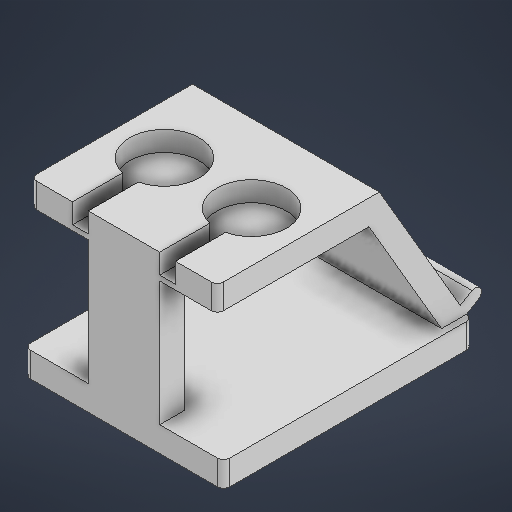
# Autodesk Inventor part: PhoneStand
Saved by Autodesk Inventor 2026.1 (Build 301233020, 233B)
## iProperties
Created: 2025-11-22
Part Number: PhoneStand
Material: Generic
Document SubType Name: Modeling
Designer: astro
Density: 1 g/cm^3
Appearance: Default
Author: astro
Autodesk Inventor part; units mm, degrees
ref_plane "YZ Plane" through (0, 0, 0) normal (1, 0, 0) x (0, 1, 0)
ref_plane "XZ Plane" through (0, 0, 0) normal (0, 1, 0) x (-1, 0, 0)
ref_plane "XY Plane" through (0, 0, 0) normal (0, 0, 1) x (1, 0, 0)
sketch "Sketch1" plane through (0, 0, 0) normal (0, 1, 0) x (-1, 0, 0)
  line L0 (-50.8, -63.5) -> (50.8, -63.5)
  line L1 (50.8, -63.5) -> (50.8, 63.5)
  line L2 (50.8, 63.5) -> (-50.8, 63.5)
  line L3 (-50.8, 63.5) -> (-50.8, -63.5)
  line L4 (-50.8, -63.5) -> (50.8, 63.5) construction
  line L5 (50.8, -63.5) -> (-50.8, 63.5) construction
  point P0 (0, 0)
  dimension "d0" = 101.6
  dimension "d1" = 127
  constraints: 12 end point, 2 midpoint, 2 parallel, 1 horizontal, 1 perpendicular
  measures "d0" distance of L2.end L1.end
  measures "d1" distance of L0.end L1.end
extrude "Extrusion1" add sketch "Sketch1" along normal blind 12.7
fillet "Fillet1" radius 3.175 4 edges at (-50.8, 6.35, 63.5) (50.8, 6.35, 63.5) (50.8, 6.35, -63.5) (-50.8, 6.35, -63.5)
sketch "Sketch2" plane through (0, 12.7, 0) normal (0, 1, 0) x (1, 0, 0)
  line L0 (47.625, 63.5) -> (-47.625, 63.5) projected
  line L1 (-47.625, 63.5) -> (47.625, 63.5)
  line L2 (47.625, 63.5) -> (47.625, 50.8)
  line L3 (47.625, 50.8) -> (-47.625, 50.8)
  line L4 (-47.625, 50.8) -> (-47.625, 63.5)
  line L5 (-47.625, -39.3448) -> (47.625, -39.3448)
  line L6 (47.625, -39.3448) -> (47.625, -60.325)
  line L7 (47.625, -60.325) -> (-47.625, -60.325)
  line L8 (-47.625, -60.325) -> (-47.625, -39.3448)
  point P0 (0, 0)
  dimension "d5" = 12.7
  constraints: 16 end point, 4 parallel, 2 horizontal, 2 perpendicular, 2 point on line
  measures "d5" distance of L1.end L2.end
extrude "Extrusion2" add sketch "Sketch2" along normal blind 76.2 contours L2 L3 L4 L0
sketch "Sketch3" plane through (47.625, 12.7, -50.8) normal (1, 0, 0) x (0, 0, -1)
  point P0 (-50.8, -12.7)
sketch "Sketch4" plane through (-47.625, 12.7, -50.8) normal (0, 0, 1) x (1, 0, 0)
  line L0 (0, 0) -> (0, 76.2) projected
  line L1 (95.25, 0) -> (98.425, 0) projected
  line L2 (0, 76.2) -> (95.25, 76.2)
  line L3 (95.25, 76.2) -> (95.25, 0)
  line L4 (95.25, 0) -> (0, 0)
  line L5 (0, 0) -> (0, 76.2)
  point P0 (47.625, -12.7)
  constraints: 8 end point, 2 parallel, 1 horizontal, 1 perpendicular
extrude "Extrusion3" add sketch "Sketch4" along normal blind 76.2
sketch "Sketch5" plane through (47.625, 12.7, -63.5) normal (1, 0, 0) x (0, 0, -1)
  line L0 (0, 76.2) -> (-88.9, 76.2) projected
  line L1 (0, 0) -> (0, 76.2) projected
  line L2 (-44.45, 76.2) -> (0, 0)
  line L3 (0, 0) -> (0, 76.2)
  line L4 (0, 76.2) -> (-44.45, 76.2)
  line L5 (0, 0) -> (-88.9, 0) projected
  line L6 (-88.9, 0) -> (-44.45, 76.2)
  line L7 (-88.9, 76.2) -> (-88.9, 0)
  line L8 (-88.9, 76.2) -> (-44.45, 76.2)
  point P0 (-63.5, -12.7)
  constraints: 12 end point, 3 perpendicular, 1 midpoint, 1 point on line
extrude "Extrusion4" cut sketch "Sketch5" against normal blind 95.25 contours L1 L2 L0
sketch "Sketch6" plane through (47.625, 12.7, 25.4) normal (1, 0, 0) x (0, 0, -1)
  line L0 (44.45, 76.2) -> (0, 76.2) projected
  line L1 (44.45, 76.2) -> (31.75, 76.2)
  line L2 (0, 0) -> (88.9, 0) projected
  line L3 (88.9, 0) -> (76.2, 0)
  line L4 (76.2, 0) -> (31.75, 76.2)
  line L5 (44.45, 76.2) -> (88.9, 0) projected
  line L6 (44.45, 76.2) -> (88.9, 0)
  line L7 (88.9, 0) -> (76.2, 0)
  line L8 (0, 76.2) -> (0, 0) projected
  line L9 (0, 76.2) -> (0, 0)
  line L10 (0, 0) -> (76.2, 0)
  line L11 (31.75, 76.2) -> (0, 76.2)
  point P0 (25.4, -12.7)
  dimension "d12" = 12.7
  dimension "d13" = 12.7
  constraints: 16 end point, 3 collinear, 2 point on line, 1 horizontal, 1 perpendicular
  measures "d12" distance of L0.start L1.end
  measures "d13" distance of L2.end L3.end
extrude "Extrusion5" cut sketch "Sketch6" against normal blind 95.25 contours L4 L2 L8 L0
sketch "Sketch7" plane through (-47.625, 12.7, -63.5) normal (-1, 0, 0) x (0, 0, 1)
  line L0 (44.45, 76.2) -> (57.15, 76.2) projected
  line L1 (127, -12.7) -> (127, 0) projected
  line L2 (57.15, 76.2) -> (127, 0)
  line L3 (57.15, 76.2) -> (127, 76.2)
  line L4 (127, 76.2) -> (127, 0)
  line L5 (57.15, 76.2) -> (12.7, 0) projected
  line L6 (49.7417, 63.5) -> (127, 63.5)
  point P0 (63.5, -12.7)
  dimension "d16" = 12.7
  constraints: 8 end point, 3 point on line, 2 perpendicular, 1 horizontal
  measures "d16" distance of L6.end L3.end
extrude "Extrusion6" add sketch "Sketch7" against normal blind 95.25 contours L3 L4 L6 L2 | L2 L6 L5
fillet "Fillet2" radius 3.175 2 edges at (47.625, 82.55, 63.5) (-47.625, 82.55, 63.5)
sketch "Sketch8" plane through (47.625, 12.7, -63.5) normal (0, 0.5039, -0.8638) x (-1, 0, 0)
  line L0 (0, 79.9133) -> (0, 6.3992) projected
  line L1 (95.25, 0) -> (0, 0) projected
  line L2 (0, 6.3992) -> (95.25, 6.3992)
  line L3 (95.25, 6.3992) -> (95.25, 0)
  line L4 (95.25, 0) -> (0, 0)
  line L5 (0, 0) -> (0, 6.3992)
  point P0 (47.625, 21.0258)
  constraints: 8 end point, 2 parallel, 1 horizontal, 1 perpendicular
extrude "Extrusion7" add sketch "Sketch8" along normal blind 10.16
fillet "Fillet3" radius 3.175 2 edges at (0, 23.3468, -69.0516) (0, 17.8193, -72.276)
sketch "Sketch9" plane through (0, 88.9, 0) normal (0, 1, 0) x (1, 0, 0)
  line L0 (-44.45, -63.5) -> (44.45, -63.5) projected
  line L1 (0, -63.5) -> (0, 19.05)
  line L2 (47.625, 19.05) -> (-47.625, 19.05) projected
  arc A0 (-47.625, -60.325) -> (-44.45, -63.5) centre (-44.45, -60.325) ccw projected
  circle A1 centre (-22.225, -20.6375) radius 17.78
  circle A2 centre (22.225, -20.6375) radius 17.78
  line L3 (-18.1992, -63.5) -> (-18.1992, -37.9557)
  line L4 (-26.2508, -37.9557) -> (-26.2508, -63.5)
  line L5 (18.1992, -37.9557) -> (18.1992, -63.5)
  line L6 (26.2508, -37.9557) -> (26.2508, -63.5)
  point P0 (0, 0)
  dimension "d23" = 35.56
  dimension "d24" = 35.56
  dimension "d25" = 8.0516
  constraints: 10 end point, 4 point on circle, 4 point on line, 2 centre point, 2 midpoint, 2 perpendicular, 1 vertical
  measures "d23" diameter of A1
  measures "d24" diameter of A2
  measures "d25" distance of L3.start L4.end
extrude "Extrusion8" cut sketch "Sketch9" against normal blind 10.16
sketch "Sketch10" plane through (-44.45, 76.2, 63.5) normal (0, 0, 1) x (1, 0, 0)
  line L0 (92.075, 0) -> (-3.175, 0) projected
  line L1 (44.45, 0) -> (44.45, -63.5)
  line L2 (92.075, -63.5) -> (-3.175, -63.5) projected
  line L3 (62.6492, 2.54) -> (62.6492, 12.7) projected
  line L4 (62.6492, 2.54) -> (62.6492, -63.5)
  line L5 (26.2508, 2.54) -> (18.1992, 2.54) projected
  line L6 (26.2508, 2.54) -> (26.2508, -63.5)
  point P0 (44.45, -76.2)
  point P1 (62.6492, 0)
  point P2 (26.2508, 0)
  constraints: 6 end point, 2 midpoint, 1 perpendicular, 1 point on line, 1 vertical
extrude "Extrusion9" add sketch "Sketch10" against normal blind 12.7
sketch "Sketch11" plane through (-47.625, 12.7, -63.5) normal (0, -0.8638, -0.5039) x (1, 0, 0)
  line L0 (95.25, -6.985) -> (0, -6.985) projected
  line L1 (47.625, -6.985) -> (47.625, 0)
  line L2 (95.25, 0) -> (0, 0) projected
  line L3 (47.625, -6.985) -> (30.101, -6.985)
  line L4 (30.101, -6.985) -> (30.101, 0)
  line L5 (47.625, -6.985) -> (65.151, -6.985)
  line L6 (65.151, -6.985) -> (65.151, 0)
  line L7 (47.625, 0) -> (30.101, 0)
  point P0 (47.625, 61.2491)
  dimension "d30" = 17.526
  constraints: 12 end point, 3 perpendicular, 3 point on line, 2 midpoint, 1 horizontal
  measures "d30" distance of L1.start L5.end
extrude "Extrusion10" cut sketch "Sketch11" against normal blind 25.4
body "Solid1"
